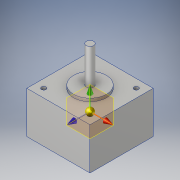
# Autodesk Inventor part: Motor
Saved by Autodesk Inventor 2018.3 (Build 223284000, 284)
## iProperties
Created: 2019-02-24
Part Number: Motor
Material: Aluminum 6061
Document SubType Name: Modeling
Designer: Mario
Mass: 4150 g
Surface Area: 98.3043 cm^2
Volume: 50.5399 cm^3
Density: 82.1133 g/cm^3
Appearance: Aluminum - Flat
Author: Mario
Autodesk Inventor part; units mm, degrees
ref_plane "YZ Plane" through (0, 0, 0) normal (1, 0, 0) x (0, 1, 0)
ref_plane "XZ Plane" through (0, 0, 0) normal (0, 1, 0) x (-1, 0, 0)
ref_plane "XY Plane" through (0, 0, 0) normal (0, 0, 1) x (1, 0, 0)
sketch "Sketch2" plane through (0, 0, 0) normal (0, 1, 0) x (-1, 0, 0)
  line L0 (-21.15, 21.15) -> (21.15, 21.15)
  line L1 (21.15, 21.15) -> (21.15, -21.15)
  line L2 (21.15, -21.15) -> (-21.15, -21.15)
  line L3 (-21.15, -21.15) -> (-21.15, 21.15)
  line L4 (-21.15, 21.15) -> (21.15, -21.15) construction
  line L5 (21.15, 21.15) -> (-21.15, -21.15) construction
  point P0 (0, 0)
  dimension "d0" = 42.3
  dimension "d1" = 42.3
  constraints: 12 end point, 2 midpoint, 2 parallel, 1 horizontal, 1 perpendicular
  measures "d0" distance of L1.end L2.end
  measures "d1" distance of L0.end L1.end
extrude "Extrusion1" add sketch "Sketch2" along normal blind 28
sketch "Sketch3" plane through (0, 28, 0) normal (0, 1, 0) x (1, 0, 0)
  circle A0 centre (0, 0) radius 11
  dimension "d4" = 22
  constraints: 1 centre point, 1 coincident
  measures "d4" diameter of A0
extrude "Extrusion2" add sketch "Sketch3" along normal blind 2
sketch "Sketch4" plane through (0, 28, 0) normal (0, 1, 0) x (1, 0, 0)
  line L0 (-24.8242, 0) -> (26.7617, 0) construction
  line L1 (0, -32.5742) -> (0, 40.8086) construction
  point P0 (0, 0)
  point P1 (-15.5, -15.5)
  point P2 (-15.5, 15.5)
  point P3 (15.5, -15.5)
  point P4 (15.5, 15.5)
  dimension "d7" = 15.5
  dimension "d8" = 15.5
  dimension "d9" = 0
  dimension "d10" = 0
  dimension "d11" = 26.7617
  dimension "d12" = 40.8086
  dimension "d13" = 32.5742
  dimension "d14" = 24.8242
  constraints: 4 end point, 3 symmetric about line, 1 horizontal, 1 vertical
  measures "d7" distance from line of point (-15.5, -15.5) L0
  measures "d8" distance from line of point (-15.5, -15.5) L1
  measures "d9" distance from line of point (0, 0) L0
  measures "d10" distance from line of point (0, 0) L1
  measures "d11" distance from line of L0.end L1
  measures "d12" distance from line of L1.end L0
  measures "d13" distance from line of L1.start L0
  measures "d14" distance from line of L0.start L1
hole "Hole1" at (-15.5, 28, 15.5) at (-15.5, 28, -15.5) at (15.5, 28, 15.5) at (15.5, 28, -15.5) direction (0, -1, 0) diameter 3 end through all
sketch "Sketch5" plane through (0, 30, 0) normal (0, 1, 0) x (1, 0, 0)
  circle A0 centre (0, 0) radius 2.5
  dimension "d22" = 5
  constraints: 1 centre point, 1 coincident
  measures "d22" diameter of A0
extrude "Extrusion3" add sketch "Sketch5" along normal blind 24
body "Solid1"
